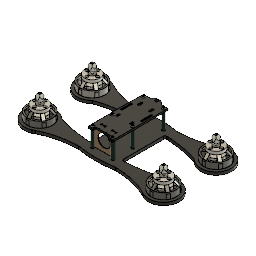
Carbon Fibre Drone Exam v2 (Autodesk Fusion 360 design; units mm, degrees)
Autodesk Fusion 360 part; units mm, degrees
note: some values were not read from the file. Chosen so that the rebuilt part matches the saved one: which bodies a step acts on; which face or edge a step refers to. Set by a fixed rule: which sketch regions a step uses.
(part 1 of 2)
sketch "Sketch1" plane through (0, 0, 0) normal (0, 1, 0) x (1, 0, 0) in component "Component"
  line L0 (50, -100) -> (-50, 100) construction
  line L1 (-50, -100) -> (50, 100) construction
  line L2 (199.7933, 69.8317) -> (-200.2067, 99.8317) construction
  line L3 (-200.2067, 69.8317) -> (199.7933, 99.8317) construction
  line L4 (-150, 0) -> (150, 0) construction
  line L5 (-200.2067, -99.8317) -> (-200.2067, -84.8317) construction
  line L6 (0, 150) -> (0, -200) construction
  spline S0 degree 5 poles (-164.8811, -49.4467) (-163.5288, -50.018) (-160.7538, -51.1452) (-156.3792, -52.7897) (-150.1158, -54.8884) (-141.5256, -57.3456) (-132.1253, -59.6259) (-121.8831, -61.7224) (-110.8317, -63.6422) (-99.042, -65.4008) (-86.5906, -67.0149) (-76.1522, -68.202) (-68.0735, -69.0377) (-62.5785, -69.571) (-59.8037, -69.8317) knots 0 0 0 0 0 0 0.1 0.2 0.3 0.4 0.5 0.6 0.7 0.8 0.9 1 1 1 1 1 1
  spline S1 degree 5 poles (-179.5589, -130.3693) (-177.6465, -129.2803) (-173.7784, -127.1456) (-167.8467, -124.0728) (-159.6742, -120.2387) (-148.9906, -115.9128) (-137.8023, -112.0905) (-126.0755, -108.8054) (-113.8059, -106.0617) (-101.0284, -103.8246) (-87.7873, -102.05) (-76.857, -100.967) (-68.4818, -100.3317) (-62.8209, -99.9855) (-59.9711, -99.8317) knots 0 0 0 0 0 0 0.1 0.2 0.3 0.4 0.5 0.6 0.7 0.8 0.9 1 1 1 1 1 1
  spline S2 degree 5 poles (-179.5589, 130.3693) (-177.6465, 129.2803) (-173.7784, 127.1456) (-167.8467, 124.0728) (-159.6742, 120.2387) (-148.9906, 115.9128) (-137.8023, 112.0905) (-126.0755, 108.8054) (-113.8059, 106.0617) (-101.0284, 103.8246) (-87.7873, 102.05) (-76.857, 100.967) (-68.4818, 100.3317) (-62.8209, 99.9855) (-59.9711, 99.8317) knots 0 0 0 0 0 0 0.1 0.2 0.3 0.4 0.5 0.6 0.7 0.8 0.9 1 1 1 1 1 1
  line L7 (-190.3068, -136.4894) -> (-168.8109, -124.2492)
  line L8 (-73.9023, -100.583) -> (-46.0398, -99.0805)
  line L9 (-190.3068, 136.4894) -> (-168.8109, 124.2492)
  line L10 (-73.9023, 100.583) -> (-46.0398, 99.0805)
  spline S3 degree 5 poles (-164.8811, 49.4467) (-163.5288, 50.018) (-160.7538, 51.1452) (-156.3792, 52.7897) (-150.1158, 54.8884) (-141.5256, 57.3456) (-132.1253, 59.6259) (-121.8831, 61.7224) (-110.8317, 63.6422) (-99.042, 65.4008) (-86.5906, 67.0149) (-76.1522, 68.202) (-68.0735, 69.0377) (-62.5785, 69.571) (-59.8037, 69.8317) knots 0 0 0 0 0 0 0.1 0.2 0.3 0.4 0.5 0.6 0.7 0.8 0.9 1 1 1 1 1 1
  line L11 (-173.4718, -45.817) -> (-156.2903, -53.0763)
  line L12 (-72.3823, -68.6499) -> (-47.2251, -71.0135)
  line L13 (-173.4718, 45.817) -> (-156.2903, 53.0763)
  line L14 (-72.3823, 68.6499) -> (-47.2251, 71.0135)
  spline S4 degree 5 poles (164.8811, 49.4467) (163.5288, 50.018) (160.7538, 51.1452) (156.3792, 52.7897) (150.1158, 54.8884) (141.5256, 57.3456) (132.1253, 59.6259) (121.8831, 61.7224) (110.8317, 63.6422) (99.042, 65.4008) (86.5906, 67.0149) (76.1522, 68.202) (68.0735, 69.0377) (62.5785, 69.571) (59.8037, 69.8317) knots 0 0 0 0 0 0 0.1 0.2 0.3 0.4 0.5 0.6 0.7 0.8 0.9 1 1 1 1 1 1
  line L15 (173.4718, 45.817) -> (156.2903, 53.0763)
  line L16 (72.3823, 68.6499) -> (47.2251, 71.0135)
  spline S5 degree 5 poles (179.5589, -130.3693) (177.6465, -129.2803) (173.7784, -127.1456) (167.8467, -124.0728) (159.6742, -120.2387) (148.9906, -115.9128) (137.8023, -112.0905) (126.0755, -108.8054) (113.8059, -106.0617) (101.0284, -103.8246) (87.7873, -102.05) (76.857, -100.967) (68.4818, -100.3317) (62.8209, -99.9855) (59.9711, -99.8317) knots 0 0 0 0 0 0 0.1 0.2 0.3 0.4 0.5 0.6 0.7 0.8 0.9 1 1 1 1 1 1
  line L17 (190.3068, -136.4894) -> (168.8109, -124.2492)
  line L18 (73.9023, -100.583) -> (46.0398, -99.0805)
  spline S6 degree 5 poles (164.8811, -49.4467) (163.5288, -50.018) (160.7538, -51.1452) (156.3792, -52.7897) (150.1158, -54.8884) (141.5256, -57.3456) (132.1253, -59.6259) (121.8831, -61.7224) (110.8317, -63.6422) (99.042, -65.4008) (86.5906, -67.0149) (76.1522, -68.202) (68.0735, -69.0377) (62.5785, -69.571) (59.8037, -69.8317) knots 0 0 0 0 0 0 0.1 0.2 0.3 0.4 0.5 0.6 0.7 0.8 0.9 1 1 1 1 1 1
  line L19 (173.4718, -45.817) -> (156.2903, -53.0763)
  line L20 (72.3823, -68.6499) -> (47.2251, -71.0135)
  spline S7 degree 5 poles (179.5589, 130.3693) (177.6465, 129.2803) (173.7784, 127.1456) (167.8467, 124.0728) (159.6742, 120.2387) (148.9906, 115.9128) (137.8023, 112.0905) (126.0755, 108.8054) (113.8059, 106.0617) (101.0284, 103.8246) (87.7873, 102.05) (76.857, 100.967) (68.4818, 100.3317) (62.8209, 99.9855) (59.9711, 99.8317) knots 0 0 0 0 0 0 0.1 0.2 0.3 0.4 0.5 0.6 0.7 0.8 0.9 1 1 1 1 1 1
  line L21 (190.3068, 136.4894) -> (168.8109, 124.2492)
  line L22 (73.9023, 100.583) -> (46.0398, 99.0805)
  spline S8 degree 5 poles (-59.9711, 99.8317) (-57.5722, 100.2237) (-52.7745, 100.9735) (-45.578, 101.9954) (-35.9826, 103.1493) (-23.9884, 104.2199) (-11.9942, 104.8857) (0, 105.1137) (11.9942, 104.8857) (23.9884, 104.2199) (35.9826, 103.1493) (45.578, 101.9954) (52.7745, 100.9735) (57.5722, 100.2237) (59.9711, 99.8317) knots 0 0 0 0 0 0 0.1 0.2 0.3 0.4 0.5 0.6 0.7 0.8 0.9 1 1 1 1 1 1
  spline S9 degree 5 poles (-59.9711, -99.8317) (-57.5722, -100.2237) (-52.7745, -100.9735) (-45.578, -101.9954) (-35.9826, -103.1493) (-23.9884, -104.2199) (-11.9942, -104.8857) (0, -105.1137) (11.9942, -104.8857) (23.9884, -104.2199) (35.9826, -103.1493) (45.578, -101.9954) (52.7745, -100.9735) (57.5722, -100.2237) (59.9711, -99.8317) knots 0 0 0 0 0 0 0.1 0.2 0.3 0.4 0.5 0.6 0.7 0.8 0.9 1 1 1 1 1 1
  line L23 (-72.1535, 97.8409) -> (-47.7886, 101.8226)
  line L24 (47.7882, 101.8225) -> (72.1539, 97.841)
  line L25 (-72.1535, -97.8409) -> (-47.7886, -101.8226)
  line L26 (47.7882, -101.8225) -> (72.1539, -97.841)
  line L27 (50, -99.8317) -> (50, -100)
  line L28 (-50, -100) -> (-50, -99.8317)
  line L29 (-50, -99.8317) -> (-49.9159, -99.8317)
  line L30 (49.9159, -99.8317) -> (50, -99.8317)
  arc A0 (-164.8811, -49.4467) -> (-173.0625, -126.8222) centre (-200.2067, -84.8317) ccw
  arc A1 (173.0625, -126.8222) -> (164.8811, -49.4467) centre (200.2067, -84.8317) ccw
  line L31 (59.8037, -69.8317) -> (55, -69.8317)
  line L32 (-55, -69.8317) -> (-59.8037, -69.8317)
  arc A2 (-173.0625, 126.8222) -> (-164.8811, 49.4467) centre (-200.2067, 84.8317) ccw
  line L33 (-50, 99.8317) -> (-49.9159, 99.8317)
  line L34 (-55, 69.8317) -> (-59.8037, 69.8317)
  line L35 (49.9159, 99.8317) -> (50, 99.8317)
  line L36 (50, 100) -> (50, 99.8317)
  line L37 (50, 64.8317) -> (50, -64.8317)
  line L38 (59.8037, 69.8317) -> (55, 69.8317)
  arc A3 (164.8811, 49.4467) -> (173.0625, 126.8221) centre (200.2067, 84.8317) ccw
  line L39 (-50, -64.8317) -> (-50, 64.8317)
  line L40 (-50, 99.8317) -> (-50, 100)
  arc A4 (-50, 64.8317) -> (-55, 69.8317) centre (-55, 64.8317) ccw
  arc A5 (-55, -69.8317) -> (-50, -64.8317) centre (-55, -64.8317) ccw
  arc A6 (50, -64.8317) -> (55, -69.8317) centre (55, -64.8317) ccw
  arc A7 (55, 69.8317) -> (50, 64.8317) centre (55, 64.8317) ccw
  point P0 (-0.2067, 84.8317)
  point P1 (-130, -60)
  point P2 (-130, -110)
  point P3 (-130, 110)
  point P4 (-130, 60)
  point P5 (130, -60)
  point P6 (130, 60)
  point P7 (130, -110)
  point P8 (130, 110)
  point P9 (0, 105)
  point P10 (0, -105)
  dimension "d1" = 100
  dimension "d2" = 200
  dimension "d3" = 400
  dimension "d4" = 30
  dimension "d5" = 15
  dimension "d6" = 100
  dimension "d7" = 5
  dimension "d8" = 5
  dimension "d9" = 5
  dimension "d10" = 5
  constraint parallel L28 L36
  constraint coincident L0 origin
  constraint coincident L1 origin
  constraint coincident L2 P0
  constraint coincident L3 P0
  constraint perpendicular L4 L36
  constraint symmetric L2.end L4 L5.start
  constraint coincident L5.end A0.centre
  constraint symmetric L4 A0 A2
  constraint symmetric L6 A0 A1
  constraint symmetric L6 A2 A3
  constraint coincident S1.start A0
  constraint midpoint S1.start L7
  constraint midpoint S1.end L8
  constraint midpoint S0.start L11
  constraint midpoint S0.end L12
  constraint symmetric L4 S0.start S3.start
  constraint symmetric L4 P1 P4
  constraint symmetric L4 S0.end S3.end
  constraint symmetric L4 S1.start S2.start
  constraint symmetric L4 P2 P3
  constraint symmetric L4 S1.end S2.end
  constraint symmetric L4 L7.start L9.start
  constraint symmetric L4 L7.end L9.end
  constraint symmetric L4 L8.start L10.start
  constraint symmetric L4 L8.end L10.end
  constraint symmetric L4 L11.start L13.start
  constraint symmetric L4 L11.end L13.end
  constraint symmetric L4 L12.start L14.start
  constraint symmetric L4 L12.end L14.end
  constraint symmetric L6 S0.start S6.start
  constraint symmetric L6 P1 P5
  constraint symmetric L6 S0.end S6.end
  constraint symmetric L6 S1.start S5.start
  constraint symmetric L6 P2 P7
  constraint symmetric L6 S1.end S5.end
  constraint symmetric L6 S2.start S7.start
  constraint symmetric L6 P3 P8
  constraint symmetric L6 S2.end S7.end
  constraint symmetric L6 L7.start L17.start
  constraint symmetric L6 L7.end L17.end
  constraint symmetric L6 L8.start L18.start
  constraint symmetric L6 L8.end L18.end
  constraint symmetric L6 L9.start L21.start
  constraint symmetric L6 L9.end L21.end
  constraint symmetric L6 L10.start L22.start
  constraint symmetric L6 L10.end L22.end
  constraint symmetric L6 S3.start S4.start
  constraint symmetric L6 P4 P6
  constraint symmetric L6 S3.end S4.end
  constraint symmetric L6 L11.start L19.start
  constraint symmetric L6 L11.end L19.end
  constraint symmetric L6 L12.start L20.start
  constraint symmetric L6 L12.end L20.end
  constraint symmetric L6 L13.start L15.start
  constraint symmetric L6 L13.end L15.end
  constraint symmetric L6 L14.start L16.start
  constraint symmetric L6 L14.end L16.end
  constraint coincident L6 P9
  constraint midpoint S2.end L23
  constraint midpoint S7.end L24
  constraint symmetric L4 S2.end S1.end
  constraint symmetric L4 S7.end S5.end
  constraint symmetric L4 P9 P10
  constraint symmetric L4 L23.start L25.start
  constraint symmetric L4 L23.end L25.end
  constraint symmetric L4 L24.start L26.start
  constraint symmetric L4 L24.end L26.end
  constraint coincident L27.start L36
  constraint collinear L27 L36
  constraint collinear L28 L39
  constraint coincident L0 L30.start
  constraint collinear L29 L30
  constraint coincident L1 L29.end
  constraint coincident S1 A0.end
  constraint coincident S5 A1.start
  constraint collinear L31 L32
  constraint coincident L1 L35.start
  constraint collinear L33 L35
  constraint coincident S2 A2.start
  constraint coincident L0 L33.end
  constraint coincident L33.start L39
  constraint collinear L36 L37
  constraint coincident S7 A3.end
  constraint collinear L39 L40
  constraint tangent L34 A4
  constraint tangent L39 A4
  constraint tangent L32 A5
  constraint tangent L39 A5
  constraint tangent L37 A6
  constraint tangent L31 A6
  constraint tangent L37 A7
  constraint tangent L38 A7
  measures "d1" distance of L0.end L1.end
  measures "d2" distance of L1.start L0.end
  measures "d3" distance of L2.end L3.end
  measures "d4" distance of L3.start L2.end
  measures "d5" distance of L5.start L5.end
  measures "d6" diameter of A0
  measures "d7" radius of A4
  measures "d8" radius of A5
  measures "d9" radius of A6
  measures "d10" radius of A7
extrude "Extrude1" add sketch "Sketch1" along normal blind 10 contours S0 S1 S2 S3 S4 S5 S6 S7 S8 S9 A0 A1 L31 L32 A2 L34 L37 L38 A3 L39 A4 A5 A6 A7 makes body 1 in component "Component"
sketch "Sketch1 (2)" plane through (0, 10, 0) normal (0, 1, 0) x (-1, 0, 0) in component "Component'"
  arc A0 (-164.8811, -49.4467) -> (-179.5589, -130.3693) centre (-200.2067, -84.8317) ccw
  spline S0 degree 5 poles (-179.5589, -130.3693) (-178.279, -129.6405) (-176.9894, -128.9214) (-175.6902, -128.2119) (-174.3812, -127.5121) (-173.0625, -126.8221) knots 0 0 0 0 0 0 0.066925 0.066925 0.066925 0.066925 0.066925 0.066925
  spline S1 degree 5 poles (-173.0625, -126.8221) (-172.4108, -126.4811) (-169.779, -125.1187) (-165.1015, -122.8003) (-158.2442, -119.6597) (-148.9906, -115.9128) (-137.8023, -112.0905) (-126.0755, -108.8054) (-113.8059, -106.0617) (-101.0284, -103.8246) (-87.7873, -102.05) (-76.857, -100.967) (-68.4818, -100.3317) (-62.8209, -99.9855) (-59.9711, -99.8317) knots 0.066925 0.066925 0.066925 0.066925 0.066925 0.066925 0.1 0.2 0.3 0.4 0.5 0.6 0.7 0.8 0.9 1 1 1 1 1 1
  spline S2 degree 5 poles (-59.9711, -99.8317) (-57.5722, -100.2237) (-52.7745, -100.9735) (-45.578, -101.9954) (-35.9826, -103.1493) (-23.9884, -104.2199) (-11.9942, -104.8857) (0, -105.1137) (11.9942, -104.8857) (23.9884, -104.2199) (35.9826, -103.1493) (45.578, -101.9954) (52.7745, -100.9735) (57.5722, -100.2237) (59.9711, -99.8317) knots -1 -1 -1 -1 -1 -1 -0.9 -0.8 -0.7 -0.6 -0.5 -0.4 -0.3 -0.2 -0.1 0 0 0 0 0 0
  spline S3 degree 5 poles (59.9711, -99.8317) (62.8209, -99.9855) (68.4818, -100.3317) (76.857, -100.967) (87.7873, -102.05) (101.0284, -103.8246) (113.8059, -106.0617) (126.0755, -108.8054) (137.8023, -112.0905) (148.9906, -115.9128) (158.2442, -119.6597) (165.1015, -122.8003) (169.779, -125.1187) (172.4108, -126.4811) (173.0625, -126.8222) knots -1 -1 -1 -1 -1 -1 -0.9 -0.8 -0.7 -0.6 -0.5 -0.4 -0.3 -0.2 -0.1 -0.066925 -0.066925 -0.066925 -0.066925 -0.066925 -0.066925
  spline S4 degree 5 poles (173.0625, -126.8222) (174.3813, -127.5122) (175.6902, -128.2119) (176.9894, -128.9214) (178.279, -129.6405) (179.5589, -130.3693) knots -0.066925 -0.066925 -0.066925 -0.066925 -0.066925 -0.066925 0 0 0 0 0 0
  arc A1 (179.5589, -130.3693) -> (164.8811, -49.4467) centre (200.2067, -84.8317) ccw
  spline S5 degree 5 poles (164.8811, -49.4467) (163.5288, -50.018) (160.7538, -51.1452) (156.3792, -52.7897) (150.1158, -54.8884) (141.5256, -57.3456) (132.1253, -59.6259) (121.8831, -61.7224) (110.8317, -63.6422) (99.042, -65.4008) (86.5906, -67.0149) (76.1522, -68.202) (68.0735, -69.0377) (62.5785, -69.571) (59.8037, -69.8317) knots 0 0 0 0 0 0 0.1 0.2 0.3 0.4 0.5 0.6 0.7 0.8 0.9 1 1 1 1 1 1
  line L0 (59.8037, -69.8317) -> (55, -69.8317)
  arc A2 (50, -64.8317) -> (55, -69.8317) centre (55, -64.8317) ccw
  line L1 (50, -64.8317) -> (50, 64.8317)
  arc A3 (55, 69.8317) -> (50, 64.8317) centre (55, 64.8317) ccw
  line L2 (55, 69.8317) -> (59.8037, 69.8317)
  spline S6 degree 5 poles (59.8037, 69.8317) (62.5785, 69.571) (68.0735, 69.0377) (76.1522, 68.202) (86.5906, 67.0149) (99.042, 65.4008) (110.8317, 63.6422) (121.8831, 61.7224) (132.1253, 59.6259) (141.5256, 57.3456) (150.1158, 54.8884) (156.3792, 52.7897) (160.7538, 51.1452) (163.5288, 50.018) (164.8811, 49.4467) knots -1 -1 -1 -1 -1 -1 -0.9 -0.8 -0.7 -0.6 -0.5 -0.4 -0.3 -0.2 -0.1 0 0 0 0 0 0
  arc A4 (164.8811, 49.4467) -> (179.5589, 130.3693) centre (200.2067, 84.8317) ccw
  spline S7 degree 5 poles (179.5589, 130.3693) (178.279, 129.6405) (176.9894, 128.9214) (175.6902, 128.2119) (174.3813, 127.5122) (173.0625, 126.8222) knots 0 0 0 0 0 0 0.066925 0.066925 0.066925 0.066925 0.066925 0.066925
  spline S8 degree 5 poles (173.0625, 126.8222) (172.4108, 126.4811) (169.779, 125.1187) (165.1015, 122.8003) (158.2442, 119.6597) (148.9906, 115.9128) (137.8023, 112.0905) (126.0755, 108.8054) (113.8059, 106.0617) (101.0284, 103.8246) (87.7873, 102.05) (76.857, 100.967) (68.4818, 100.3317) (62.8209, 99.9855) (59.9711, 99.8317) knots 0.066925 0.066925 0.066925 0.066925 0.066925 0.066925 0.1 0.2 0.3 0.4 0.5 0.6 0.7 0.8 0.9 1 1 1 1 1 1
  spline S9 degree 5 poles (59.9711, 99.8317) (57.5722, 100.2237) (52.7745, 100.9735) (45.578, 101.9954) (35.9826, 103.1493) (23.9884, 104.2199) (11.9942, 104.8857) (0, 105.1137) (-11.9942, 104.8857) (-23.9884, 104.2199) (-35.9826, 103.1493) (-45.578, 101.9954) (-52.7745, 100.9735) (-57.5722, 100.2237) (-59.9711, 99.8317) knots 0 0 0 0 0 0 0.1 0.2 0.3 0.4 0.5 0.6 0.7 0.8 0.9 1 1 1 1 1 1
  spline S10 degree 5 poles (-59.9711, 99.8317) (-62.8209, 99.9855) (-68.4818, 100.3317) (-76.857, 100.967) (-87.7873, 102.05) (-101.0284, 103.8246) (-113.8059, 106.0617) (-126.0755, 108.8054) (-137.8023, 112.0905) (-148.9906, 115.9128) (-158.2442, 119.6597) (-165.1015, 122.8003) (-169.779, 125.1187) (-172.4108, 126.4811) (-173.0625, 126.8222) knots -1 -1 -1 -1 -1 -1 -0.9 -0.8 -0.7 -0.6 -0.5 -0.4 -0.3 -0.2 -0.1 -0.066925 -0.066925 -0.066925 -0.066925 -0.066925 -0.066925
  spline S11 degree 5 poles (-173.0625, 126.8222) (-174.3813, 127.5122) (-175.6902, 128.2119) (-176.9894, 128.9214) (-178.279, 129.6405) (-179.5589, 130.3693) knots -0.066925 -0.066925 -0.066925 -0.066925 -0.066925 -0.066925 0 0 0 0 0 0
  arc A5 (-179.5589, 130.3693) -> (-164.8811, 49.4467) centre (-200.2067, 84.8317) ccw
  spline S12 degree 5 poles (-164.8811, 49.4467) (-163.5288, 50.018) (-160.7538, 51.1452) (-156.3792, 52.7897) (-150.1158, 54.8884) (-141.5256, 57.3456) (-132.1253, 59.6259) (-121.8831, 61.7224) (-110.8317, 63.6422) (-99.042, 65.4008) (-86.5906, 67.0149) (-76.1522, 68.202) (-68.0735, 69.0377) (-62.5785, 69.571) (-59.8037, 69.8317) knots 0 0 0 0 0 0 0.1 0.2 0.3 0.4 0.5 0.6 0.7 0.8 0.9 1 1 1 1 1 1
  line L3 (-59.8037, 69.8317) -> (-55, 69.8317)
  arc A6 (-50, 64.8317) -> (-55, 69.8317) centre (-55, 64.8317) ccw
  line L4 (-50, 64.8317) -> (-50, -64.8317)
  arc A7 (-55, -69.8317) -> (-50, -64.8317) centre (-55, -64.8317) ccw
  line L5 (-55, -69.8317) -> (-59.8037, -69.8317)
  spline S13 degree 5 poles (-59.8037, -69.8317) (-62.5785, -69.571) (-68.0735, -69.0377) (-76.1522, -68.202) (-86.5906, -67.0149) (-99.042, -65.4008) (-110.8317, -63.6422) (-121.8831, -61.7224) (-132.1253, -59.6259) (-141.5256, -57.3456) (-150.1158, -54.8884) (-156.3792, -52.7897) (-160.7538, -51.1452) (-163.5288, -50.018) (-164.8811, -49.4467) knots -1 -1 -1 -1 -1 -1 -0.9 -0.8 -0.7 -0.6 -0.5 -0.4 -0.3 -0.2 -0.1 0 0 0 0 0 0
  line L6 (40, 88) -> (40, -90)
  line L7 (-40, -90) -> (-40, 88)
  line L8 (-40, 90) -> (40, -90) construction
  line L9 (40, 90) -> (-40, -90) construction
  line L10 (23, 79.4003) -> (-23, 79.4003)
  line L11 (-25, 81.4003) -> (-25, 88)
  line L12 (25, 88) -> (25, 81.4003)
  circle A8 centre (33, 82) radius 5
  line L13 (-38, 90) -> (-27, 90)
  line L14 (27, 90) -> (38, 90)
  arc A9 (23, 79.4003) -> (25, 81.4003) centre (23, 81.4003) ccw
  arc A10 (27, 90) -> (25, 88) centre (27, 88) ccw
  arc A11 (40, 88) -> (38, 90) centre (38, 88) ccw
  arc A12 (-25, 81.4003) -> (-23, 79.4003) centre (-23, 81.4003) ccw
  arc A13 (-25, 88) -> (-27, 90) centre (-27, 88) ccw
  arc A14 (-38, 90) -> (-40, 88) centre (-38, 88) ccw
  line L15 (0, 0) -> (0, 150)
  line L16 (0, 150) -> (0, 0)
  line L17 (0, 0) -> (0, -150)
  circle A15 centre (-33, 82) radius 5
  line L18 (150, 0) -> (-150, 0)
  line L19 (150, 50) -> (-150, 50)
  circle A16 centre (33, 18) radius 5
  circle A17 centre (-33, 18) radius 5
  circle A18 centre (33, -82) radius 5
  circle A19 centre (-33, -82) radius 5
  line L20 (11.2, 59) -> (10.8383, 59)
  line L21 (10.0383, 59.8) -> (10.0383, 64.2284)
  line L22 (10.8383, 65.0284) -> (11.2, 65.0284)
  line L23 (24, 59.2) -> (24.0338, 59.2)
  line L24 (24.0338, 65.0284) -> (24, 65.0284)
  line L25 (24.8, 64.2284) -> (24.8, 60)
  line L26 (23.2338, 61.1579) -> (12, 61.1579)
  line L27 (12, 63.1245) -> (23.2338, 63.1245)
  line L28 (23.2338, 60) -> (23.2338, 61.1579)
  line L29 (23.2338, 63.1245) -> (23.2338, 64.2284)
  line L30 (12, 64.2284) -> (12, 63.1245)
  line L31 (12, 61.1579) -> (12, 59.8)
  arc A20 (23.2338, 60) -> (24.0338, 59.2) centre (24.0338, 60) ccw
  arc A21 (24, 59.2) -> (24.8, 60) centre (24, 60) ccw
  arc A22 (24.8, 64.2284) -> (24, 65.0284) centre (24, 64.2284) ccw
  arc A23 (24.0338, 65.0284) -> (23.2338, 64.2284) centre (24.0338, 64.2284) ccw
  arc A24 (11.2, 59) -> (12, 59.8) centre (11.2, 59.8) ccw
  arc A25 (10.0383, 59.8) -> (10.8383, 59) centre (10.8383, 59.8) ccw
  arc A26 (12, 64.2284) -> (11.2, 65.0284) centre (11.2, 64.2284) ccw
  arc A27 (10.8383, 65.0284) -> (10.0383, 64.2284) centre (10.8383, 64.2284) ccw
  line L32 (18.3125, -64.8317) -> (18, -64.8317)
  line L33 (15, -61.8317) -> (15, -53)
  line L34 (18, -50) -> (18.3125, -50)
  line L35 (21.3125, -53) -> (21.3125, -61.8317)
  line L36 (35, -45) -> (30, -45)
  line L37 (30, -45) -> (30, -10)
  line L38 (30, -10) -> (35, -10)
  line L39 (35, -10) -> (35, -45)
  arc A28 (15, -61.8317) -> (18, -64.8317) centre (18, -61.8317) ccw
  arc A29 (18.3125, -64.8317) -> (21.3125, -61.8317) centre (18.3125, -61.8317) ccw
  arc A30 (21.3125, -53) -> (18.3125, -50) centre (18.3125, -53) ccw
  arc A31 (18, -50) -> (15, -53) centre (18, -53) ccw
  line L40 (-30, -45) -> (-30, -10)
  line L41 (-35, -10) -> (-35, -45)
  line L42 (-35, -45) -> (-30, -45)
  line L43 (-30, -10) -> (-35, -10)
  line L44 (-15, -61.8317) -> (-15, -53)
  arc A32 (-15, -53) -> (-18, -50) centre (-18, -53) ccw
  arc A33 (-18.3125, -50) -> (-21.3125, -53) centre (-18.3125, -53) ccw
  line L45 (-21.3125, -53) -> (-21.3125, -61.8317)
  arc A34 (-21.3125, -61.8317) -> (-18.3125, -64.8317) centre (-18.3125, -61.8317) ccw
  arc A35 (-18, -64.8317) -> (-15, -61.8317) centre (-18, -61.8317) ccw
  line L46 (-18.3125, -64.8317) -> (-18, -64.8317)
  line L47 (-18, -50) -> (-18.3125, -50)
  line L48 (-12, 63.1245) -> (-23.2338, 63.1245)
  line L49 (-23.2338, 61.1579) -> (-12, 61.1579)
  line L50 (-24.8, 64.2284) -> (-24.8, 60)
  arc A36 (-23.2338, 64.2284) -> (-24.0338, 65.0284) centre (-24.0338, 64.2284) ccw
  arc A37 (-24, 65.0284) -> (-24.8, 64.2284) centre (-24, 64.2284) ccw
  line L51 (-23.2338, 63.1245) -> (-23.2338, 64.2284)
  line L52 (-23.2338, 60) -> (-23.2338, 61.1579)
  arc A38 (-24.8, 60) -> (-24, 59.2) centre (-24, 60) ccw
  arc A39 (-24.0338, 59.2) -> (-23.2338, 60) centre (-24.0338, 60) ccw
  line L53 (-10.0383, 59.8) -> (-10.0383, 64.2284)
  line L54 (-12, 64.2284) -> (-12, 63.1245)
  arc A40 (-11.2, 65.0284) -> (-12, 64.2284) centre (-11.2, 64.2284) ccw
  line L55 (-12, 61.1579) -> (-12, 59.8)
  arc A41 (-12, 59.8) -> (-11.2, 59) centre (-11.2, 59.8) ccw
  line L56 (-11.2, 59) -> (-10.8383, 59)
  arc A42 (-10.8383, 59) -> (-10.0383, 59.8) centre (-10.8383, 59.8) ccw
  arc A43 (-10.0383, 64.2284) -> (-10.8383, 65.0284) centre (-10.8383, 64.2284) ccw
  line L57 (-10.8383, 65.0284) -> (-11.2, 65.0284)
  line L58 (25, 5) -> (20, 5)
  line L59 (20, 5) -> (20, 15)
  line L60 (20, 15) -> (25, 15)
  line L61 (25, 15) -> (25, 5)
  line L62 (-20, 5) -> (-20, 15)
  line L63 (-25, 5) -> (-20, 5)
  line L64 (-25, 15) -> (-25, 5)
  line L65 (-20, 15) -> (-25, 15)
  arc A44 (-16.3, -92.0308) -> (16.3, -92.0308) centre (0, -80) ccw
  line L66 (40, -90) -> (20.3229, -90)
  line L67 (-20.3229, -90) -> (-40, -90)
  arc A45 (20.3229, -90) -> (16.3, -92.0308) centre (20.3229, -95) ccw
  arc A46 (-16.3, -92.0308) -> (-20.3229, -90) centre (-20.3229, -95) ccw
  circle A47 centre (0, -93.2666) radius 5
  point P0 (-33, -82)
  dimension "d13" = 10
  dimension "d14" = 2
  dimension "d15" = 2
  dimension "d16" = 2
  dimension "d17" = 2
  dimension "d18" = 2
  dimension "d19" = 2
  dimension "d20" = 10
  dimension "d21" = 0.8
  dimension "d22" = 0.8
  dimension "d23" = 0.8
  dimension "d24" = 0.8
  dimension "d25" = 0.8
  dimension "d26" = 0.8
  dimension "d27" = 0.8
  dimension "d28" = 0.8
  dimension "d29" = 3
  dimension "d30" = 3
  dimension "d31" = 3
  dimension "d32" = 3
  dimension "d33" = 5
  dimension "d34" = 5
  dimension "d37" = 10
  constraint horizontal L13
  constraint perpendicular L6 L13
  constraint parallel L13 L66
  constraint parallel L6 L7
  constraint coincident L8 L15.start
  constraint coincident L9 L15.start
  constraint coincident L15.start L16.end
  constraint horizontal L10
  constraint vertical L11
  constraint vertical L12
  constraint collinear L13 L14
  constraint tangent L12 A9
  constraint tangent L10 A9
  constraint tangent L12 A10
  constraint tangent L14 A10
  constraint coincident L9.start L6
  constraint coincident L9.start L14
  constraint tangent L6 A11
  constraint tangent L14 A11
  constraint tangent L10 A12
  constraint tangent L11 A12
  constraint tangent L11 A13
  constraint tangent L13 A13
  constraint coincident L8.start L13
  constraint coincident L8.start L7
  constraint tangent L13 A14
  constraint tangent L7 A14
  constraint perpendicular L10 L15
  constraint parallel L15 L16
  constraint perpendicular L17 L66
  constraint symmetric A8 L16 A15
  constraint perpendicular L4 L18
  constraint perpendicular L4 L19
  constraint symmetric A8 L19 A16
  constraint symmetric A15 L19 A17
  constraint symmetric A8 L18 A18
  constraint symmetric A15.centre L18 P0
  constraint coincident P0 A19.centre
  constraint coincident L17 A44.centre
  constraint horizontal L27
  constraint horizontal L20
  constraint vertical L21
  constraint horizontal L22
  constraint vertical L30
  constraint horizontal L23
  constraint vertical L28
  constraint horizontal L24
  constraint vertical L25
  constraint coincident L27.end L28
  constraint collinear L28 L29
  constraint collinear L30 L31
  constraint tangent L28 A20
  constraint tangent L23 A20
  constraint tangent L23 A21
  constraint tangent L25 A21
  constraint tangent L25 A22
  constraint tangent L24 A22
  constraint tangent L29 A23
  constraint tangent L24 A23
  constraint tangent L31 A24
  constraint tangent L20 A24
  constraint tangent L21 A25
  constraint tangent L20 A25
  constraint tangent L30 A26
  constraint tangent L22 A26
  constraint tangent L22 A27
  constraint tangent L21 A27
  constraint horizontal L32
  constraint vertical L33
  constraint horizontal L34
  constraint vertical L35
  constraint horizontal L36
  constraint vertical L37
  constraint horizontal L38
  constraint vertical L39
  constraint tangent L32 A28
  constraint tangent L33 A28
  constraint tangent L32 A29
  constraint tangent L35 A29
  constraint tangent L35 A30
  constraint tangent L34 A30
  constraint tangent L33 A31
  constraint tangent L34 A31
  constraint symmetric L15 L26.start L49.start
  constraint symmetric L15 L27.end L48.end
  constraint symmetric L15 L27.start L48.start
  constraint symmetric L15 L26.end L49.end
  constraint symmetric L15 L28.start L52.start
  constraint symmetric L15 L23.end A39.start
  constraint symmetric L15 A20 A39
  constraint symmetric L15 L23.start A38.end
  constraint symmetric L15 L25.end L50.end
  constraint symmetric L15 A21 A38
  constraint symmetric L15 L25.start L50.start
  constraint symmetric L15 L24.end A37.start
  constraint symmetric L15 A22 A37
  constraint symmetric L15 L29.end A36.start
  constraint symmetric L15 L24.start A36.end
  constraint symmetric L15 A23 A36
  constraint symmetric L15 L31.end L55.end
  constraint symmetric L15 L20.start A41.end
  constraint symmetric L15 A24 A41
  constraint symmetric L15 L21.start L53.start
  constraint symmetric L15 L20.end L56.end
  constraint symmetric L15 A25 A42
  constraint symmetric L15 L30.start L54.start
  constraint symmetric L15 L22.end A40.start
  constraint symmetric L15 A26 A40
  constraint symmetric L15 L22.start A43.end
  constraint symmetric L15 L21.end L53.end
  constraint symmetric L15 A27 A43
  constraint symmetric L15 L36.start L41.end
  constraint symmetric L15 L36.end L40.start
  constraint symmetric L15 L37.end L40.end
  constraint symmetric L15 L38.end L41.start
  constraint symmetric L15 L32.end A35.start
  constraint symmetric L15 L33.start L44.start
  constraint symmetric L15 A28 A35
  constraint symmetric L15 L32.start A34.end
  constraint symmetric L15 L35.end L45.end
  constraint symmetric L15 A29 A34
  constraint symmetric L15 L35.start A33.end
  constraint symmetric L15 L34.end A33.start
  constraint symmetric L15 A30 A33
  constraint symmetric L15 L33.end L44.end
  constraint symmetric L15 L34.start A32.end
  constraint symmetric L15 A31 A32
  constraint horizontal L58
  constraint vertical L59
  constraint horizontal L60
  constraint vertical L61
  constraint symmetric L15 L58.start L63.start
  constraint symmetric L15 L58.end L62.start
  constraint symmetric L15 L59.end L62.end
  constraint symmetric L15 L60.end L64.start
  constraint collinear L66 L67
  constraint tangent L66 A45
  constraint tangent A44 A45
  constraint tangent A44 A46
  constraint tangent L67 A46
  constraint coincident L17 A47.centre
  measures "d13" diameter of A8
  measures "d14" radius of A9
  measures "d15" radius of A10
  measures "d16" radius of A11
  measures "d17" radius of A12
  measures "d18" radius of A13
  measures "d19" radius of A14
  measures "d20" diameter of A19
  measures "d21" radius of A20
  measures "d22" radius of A21
  measures "d23" radius of A22
  measures "d24" radius of A23
  measures "d25" radius of A24
  measures "d26" radius of A25
  measures "d27" radius of A26
  measures "d28" radius of A27
  measures "d29" radius of A28
  measures "d30" radius of A29
  measures "d31" radius of A30
  measures "d32" radius of A31
  measures "d33" radius of A45
  measures "d34" radius of A46
  measures "d37" diameter of A47
extrude "Extrude2" add sketch "Sketch1 (2)" along normal blind 58 separate body contours L20 L21 L22 L23 L24 L25 L26 L27 L28 L29 L30 L31 A20 A21 A22 A23 A24 A25 A26 A27 | L36 L37 L38 L39 | L40 L41 L42 L43 | L48 L49 L50 A36 A37 L51 L52 A38 A39 L53 L54 A40 L55 A41 L56 A42 A43 L57 | L58 L59 L60 L61 | L62 L63 L64 L65 makes body 2 at (25, 48.6667, 11.6667) makes body 3 at (19.4892, 29.3333, 61.1579) makes body 4 at (-30, 29.3333, -33.3333) makes body 5 at (-20, 48.6667, 8.3333) makes body 6 at (-19.4892, 29.3333, 61.1579) makes body 7 at (35, 29.3333, -21.6667) in component "Component'"
extrude "Extrude1'" add sketch "Sketch1 (2)" along normal blind 60 separate body contours L7 L17 L18 A44 L67 A46 A47 | L6 L17 L18 A44 L66 A45 A47 | L7 L15 L16 L18 L19 | L7 L10 L11 L13 A12 A13 A14 L15 L16 L19 | L6 L15 L16 L18 L19 | L6 L10 L12 L14 A9 A10 A11 L15 L16 L19 makes body 8 in component "Component'"
sketch "Sketch2" plane through (40, 0, 0) normal (1, 0, 0) x (0, 0, -1) in component "Component'"
  line L0 (-88, 10) -> (90, 10)
  line L1 (90, 10) -> (90, 70)
  line L2 (90, 70) -> (-88, 70)
  line L3 (-88, 70) -> (-88, 10)
  line L4 (-95.3524, 10) -> (104.6476, 10)
  line L5 (104.6476, 10) -> (104.6476, 65)
  line L6 (104.6476, 65) -> (-95.3524, 65)
  line L7 (-95.3524, 65) -> (-95.3524, 10)
  dimension "d40" = 200
  dimension "d41" = 55
  constraint horizontal L4
  constraint vertical L5
  constraint horizontal L6
  constraint vertical L7
  measures "d40" distance of L4.start L4.end
  measures "d41" distance of L4.start L6.end
extrude "Extrude3" cut sketch "Sketch2" against normal blind 120 contours L0 L1 L3 L4 L6 | L3 L4 L6 L7 | L1 L4 L5 L6 bodies 2 3 4 5 6 7 8 in component "Component'"
extrude "Extrude4" add sketch "Sketch1 (2)" along normal blind 60 separate body contours A8 | A15 | A16 | A17 | A18 | A19 makes body 9 at (28.0248, 50, -82.4978) makes body 10 at (36.8302, 50, 78.7861) makes body 11 at (-37.9752, 50, 17.5022) makes body 12 at (28.0248, 50, 17.5022) makes body 13 at (-29.5088, 50, 85.5793) makes body 14 at (-29.5088, 50, -78.4207) in component "Component'"
ref_plane "WorkPlane1" through (0, 67.5, 75.4003) normal (0, 0, 1) x (1, 0, 0) in component "Component'"
sketch "Sketch4" plane through (0, 67.5, 75.4003) normal (0, 0, 1) x (1, 0, 0) in component "Component'"
  line L0 (-33, 0) -> (32.8247, 0)
  line L1 (32.8247, 0) -> (32.8247, -57.541)
  line L2 (32.8247, -57.541) -> (-33, -57.541)
  line L3 (-33, -57.541) -> (-33, 0)
  circle A0 centre (0, -25) radius 20
  dimension "d47" = 40
  constraint horizontal L0
  constraint vertical L1
  constraint horizontal L2
  constraint vertical L3
  measures "d47" diameter of A0
extrude "Extrude5" add sketch "Sketch4" along normal blind 1.6 separate body makes body 15 in component "Component'"
sketch "Sketch5" plane through (0, 70, 0) normal (0, 1, 0) x (-1, 0, 0) in component "Component'"
  circle A0 centre (33, 82) radius 5
  circle A1 centre (33, 82) radius 5.5
  circle A2 centre (33, 82) radius 1
  spline S0 degree 5 poles (33.8119, 81.4162) (33.7795, 81.233) (33.7145, 80.8824) (33.6171, 80.4047) (33.4872, 79.8652) (33.3248, 79.3647) (33.1624, 79.0534) (33, 78.9469) (32.8376, 79.0534) (32.6752, 79.3647) (32.5128, 79.8652) (32.3829, 80.4047) (32.2855, 80.8824) (32.2206, 81.233) (32.1881, 81.4162) knots 0 0 0 0 0 0 0.1 0.2 0.3 0.4 0.5 0.6 0.7 0.8 0.9 1 1 1 1 1 1
  spline S1 degree 5 poles (33.5838, 82.8119) (33.767, 82.7795) (34.1176, 82.7145) (34.5953, 82.6171) (35.1348, 82.4872) (35.6353, 82.3248) (35.9466, 82.1624) (36.0531, 82) (35.9466, 81.8376) (35.6353, 81.6752) (35.1348, 81.5128) (34.5953, 81.3829) (34.1176, 81.2855) (33.767, 81.2206) (33.5838, 81.1881) knots 0 0 0 0 0 0 0.1 0.2 0.3 0.4 0.5 0.6 0.7 0.8 0.9 1 1 1 1 1 1
  spline S2 degree 5 poles (32.1881, 82.5838) (32.2206, 82.767) (32.2855, 83.1176) (32.3829, 83.5953) (32.5128, 84.1348) (32.6752, 84.6353) (32.8376, 84.9466) (33, 85.0531) (33.1624, 84.9466) (33.3248, 84.6353) (33.4872, 84.1348) (33.6171, 83.5953) (33.7145, 83.1176) (33.7795, 82.767) (33.8119, 82.5838) knots 0 0 0 0 0 0 0.1 0.2 0.3 0.4 0.5 0.6 0.7 0.8 0.9 1 1 1 1 1 1
  spline S3 degree 5 poles (32.4162, 81.1881) (32.233, 81.2206) (31.8824, 81.2855) (31.4047, 81.3829) (30.8652, 81.5128) (30.3647, 81.6752) (30.0534, 81.8376) (29.9469, 82) (30.0534, 82.1624) (30.3647, 82.3248) (30.8652, 82.4872) (31.4047, 82.6171) (31.8824, 82.7145) (32.233, 82.7795) (32.4162, 82.8119) knots 0 0 0 0 0 0 0.1 0.2 0.3 0.4 0.5 0.6 0.7 0.8 0.9 1 1 1 1 1 1
  point P0 (33, 79)
  point P1 (36, 82)
  point P2 (33, 85)
  point P3 (30, 82)
  dimension "d50" = 11
  dimension "d51" = 2
  dimension "d53" = 360
  constraint concentric A0 A1
  constraint concentric A0 A2
  constraint coincident A2 S0.start
  constraint coincident A2 S0.end
  measures "d50" diameter of A1
  measures "d51" diameter of A2
extrude "Extrude7" add sketch "Sketch5" along normal blind 2 separate body contours A0 | A1 makes body 16 in component "Component'"
extrude "Extrude6" add sketch "Sketch5" along normal blind 2 separate body contours A0 | A1 | A2 S0 S1 S2 | A2 S1 S2 S3 | A2 S0 S1 S3 | A2 S0 S2 S3 makes body 17 in component "Component'"
extrude "Extrude8" add 1 faces at (-35.0904, 72, 79.8056) along direction (0, 1, 0) blind 1 on bodies 16 bodies 16 17 in component "Component'"
extrude "Extrude9" add sketch "Sketch5" along normal blind 1 separate body contours A2 makes body 18 in component "Component'"
fillet "Fillet1" radius 1.5 1 faces at (-38.4727, 71, 81.4524) on bodies 16 in component "Component'"
mirror "Mirror1" about plane through (0, 0, 0) normal (1, 0, 0) of bodies 18 16 makes body 19 at (27.6963, 71.7841, 80.6495) makes body 20 at (32.5256, 70, 81.7774) in component "Component'"
mirror "Mirror2" about plane through (0, 0, 0) normal (0, 0, 1) of bodies 19 16 20 makes body 21 at (-27.6963, 71.7841, -80.6495) makes body 22 at (27.6963, 71.7841, -80.6495) makes body 23 at (32.5256, 70, -81.7774) in component "Component'"
copy_body "CopyPasteBodies1" bodies 18 19 16 makes body 24 makes body 25 makes body 26 in component "Component'"
move_body "Move1" bodies 24 25 26 to x (1, 0, 0) y (0, 1, 0) z (0, 0, 1) at (0, 0, -64) in component "Component'"
sketch "Sketch1 (3)" plane through (0, 10, 0) normal (0, 1, 0) x (-1, 0, 0) in component "Component''"
  arc A0 (-164.8811, -49.4467) -> (-179.5589, -130.3693) centre (-200.2067, -84.8317) ccw
  spline S0 degree 5 poles (-179.5589, -130.3693) (-178.279, -129.6405) (-176.9894, -128.9214) (-175.6902, -128.2119) (-174.3812, -127.5121) (-173.0625, -126.8221) knots 0 0 0 0 0 0 0.066925 0.066925 0.066925 0.066925 0.066925 0.066925
  spline S1 degree 5 poles (-173.0625, -126.8221) (-172.4108, -126.4811) (-169.779, -125.1187) (-165.1015, -122.8003) (-158.2442, -119.6597) (-148.9906, -115.9128) (-137.8023, -112.0905) (-126.0755, -108.8054) (-113.8059, -106.0617) (-101.0284, -103.8246) (-87.7873, -102.05) (-76.857, -100.967) (-68.4818, -100.3317) (-62.8209, -99.9855) (-59.9711, -99.8317) knots 0.066925 0.066925 0.066925 0.066925 0.066925 0.066925 0.1 0.2 0.3 0.4 0.5 0.6 0.7 0.8 0.9 1 1 1 1 1 1
  spline S2 degree 5 poles (-59.9711, -99.8317) (-57.5722, -100.2237) (-52.7745, -100.9735) (-45.578, -101.9954) (-35.9826, -103.1493) (-23.9884, -104.2199) (-11.9942, -104.8857) (0, -105.1137) (11.9942, -104.8857) (23.9884, -104.2199) (35.9826, -103.1493) (45.578, -101.9954) (52.7745, -100.9735) (57.5722, -100.2237) (59.9711, -99.8317) knots -1 -1 -1 -1 -1 -1 -0.9 -0.8 -0.7 -0.6 -0.5 -0.4 -0.3 -0.2 -0.1 0 0 0 0 0 0
  spline S3 degree 5 poles (59.9711, -99.8317) (62.8209, -99.9855) (68.4818, -100.3317) (76.857, -100.967) (87.7873, -102.05) (101.0284, -103.8246) (113.8059, -106.0617) (126.0755, -108.8054) (137.8023, -112.0905) (148.9906, -115.9128) (158.2442, -119.6597) (165.1015, -122.8003) (169.779, -125.1187) (172.4108, -126.4811) (173.0625, -126.8222) knots -1 -1 -1 -1 -1 -1 -0.9 -0.8 -0.7 -0.6 -0.5 -0.4 -0.3 -0.2 -0.1 -0.066925 -0.066925 -0.066925 -0.066925 -0.066925 -0.066925
  spline S4 degree 5 poles (173.0625, -126.8222) (174.3813, -127.5122) (175.6902, -128.2119) (176.9894, -128.9214) (178.279, -129.6405) (179.5589, -130.3693) knots -0.066925 -0.066925 -0.066925 -0.066925 -0.066925 -0.066925 0 0 0 0 0 0
  arc A1 (179.5589, -130.3693) -> (164.8811, -49.4467) centre (200.2067, -84.8317) ccw
  spline S5 degree 5 poles (164.8811, -49.4467) (163.5288, -50.018) (160.7538, -51.1452) (156.3792, -52.7897) (150.1158, -54.8884) (141.5256, -57.3456) (132.1253, -59.6259) (121.8831, -61.7224) (110.8317, -63.6422) (99.042, -65.4008) (86.5906, -67.0149) (76.1522, -68.202) (68.0735, -69.0377) (62.5785, -69.571) (59.8037, -69.8317) knots 0 0 0 0 0 0 0.1 0.2 0.3 0.4 0.5 0.6 0.7 0.8 0.9 1 1 1 1 1 1
  line L0 (59.8037, -69.8317) -> (55, -69.8317)
  arc A2 (50, -64.8317) -> (55, -69.8317) centre (55, -64.8317) ccw
  line L1 (50, -64.8317) -> (50, 64.8317)
  arc A3 (55, 69.8317) -> (50, 64.8317) centre (55, 64.8317) ccw
  line L2 (55, 69.8317) -> (59.8037, 69.8317)
  spline S6 degree 5 poles (59.8037, 69.8317) (62.5785, 69.571) (68.0735, 69.0377) (76.1522, 68.202) (86.5906, 67.0149) (99.042, 65.4008) (110.8317, 63.6422) (121.8831, 61.7224) (132.1253, 59.6259) (141.5256, 57.3456) (150.1158, 54.8884) (156.3792, 52.7897) (160.7538, 51.1452) (163.5288, 50.018) (164.8811, 49.4467) knots -1 -1 -1 -1 -1 -1 -0.9 -0.8 -0.7 -0.6 -0.5 -0.4 -0.3 -0.2 -0.1 0 0 0 0 0 0
  arc A4 (164.8811, 49.4467) -> (179.5589, 130.3693) centre (200.2067, 84.8317) ccw
  spline S7 degree 5 poles (179.5589, 130.3693) (178.279, 129.6405) (176.9894, 128.9214) (175.6902, 128.2119) (174.3813, 127.5122) (173.0625, 126.8222) knots 0 0 0 0 0 0 0.066925 0.066925 0.066925 0.066925 0.066925 0.066925
  spline S8 degree 5 poles (173.0625, 126.8222) (172.4108, 126.4811) (169.779, 125.1187) (165.1015, 122.8003) (158.2442, 119.6597) (148.9906, 115.9128) (137.8023, 112.0905) (126.0755, 108.8054) (113.8059, 106.0617) (101.0284, 103.8246) (87.7873, 102.05) (76.857, 100.967) (68.4818, 100.3317) (62.8209, 99.9855) (59.9711, 99.8317) knots 0.066925 0.066925 0.066925 0.066925 0.066925 0.066925 0.1 0.2 0.3 0.4 0.5 0.6 0.7 0.8 0.9 1 1 1 1 1 1
  spline S9 degree 5 poles (59.9711, 99.8317) (57.5722, 100.2237) (52.7745, 100.9735) (45.578, 101.9954) (35.9826, 103.1493) (23.9884, 104.2199) (11.9942, 104.8857) (0, 105.1137) (-11.9942, 104.8857) (-23.9884, 104.2199) (-35.9826, 103.1493) (-45.578, 101.9954) (-52.7745, 100.9735) (-57.5722, 100.2237) (-59.9711, 99.8317) knots 0 0 0 0 0 0 0.1 0.2 0.3 0.4 0.5 0.6 0.7 0.8 0.9 1 1 1 1 1 1
  spline S10 degree 5 poles (-59.9711, 99.8317) (-62.8209, 99.9855) (-68.4818, 100.3317) (-76.857, 100.967) (-87.7873, 102.05) (-101.0284, 103.8246) (-113.8059, 106.0617) (-126.0755, 108.8054) (-137.8023, 112.0905) (-148.9906, 115.9128) (-158.2442, 119.6597) (-165.1015, 122.8003) (-169.779, 125.1187) (-172.4108, 126.4811) (-173.0625, 126.8222) knots -1 -1 -1 -1 -1 -1 -0.9 -0.8 -0.7 -0.6 -0.5 -0.4 -0.3 -0.2 -0.1 -0.066925 -0.066925 -0.066925 -0.066925 -0.066925 -0.066925
  spline S11 degree 5 poles (-173.0625, 126.8222) (-174.3813, 127.5122) (-175.6902, 128.2119) (-176.9894, 128.9214) (-178.279, 129.6405) (-179.5589, 130.3693) knots -0.066925 -0.066925 -0.066925 -0.066925 -0.066925 -0.066925 0 0 0 0 0 0
  arc A5 (-179.5589, 130.3693) -> (-164.8811, 49.4467) centre (-200.2067, 84.8317) ccw
  spline S12 degree 5 poles (-164.8811, 49.4467) (-163.5288, 50.018) (-160.7538, 51.1452) (-156.3792, 52.7897) (-150.1158, 54.8884) (-141.5256, 57.3456) (-132.1253, 59.6259) (-121.8831, 61.7224) (-110.8317, 63.6422) (-99.042, 65.4008) (-86.5906, 67.0149) (-76.1522, 68.202) (-68.0735, 69.0377) (-62.5785, 69.571) (-59.8037, 69.8317) knots 0 0 0 0 0 0 0.1 0.2 0.3 0.4 0.5 0.6 0.7 0.8 0.9 1 1 1 1 1 1
  line L3 (-59.8037, 69.8317) -> (-55, 69.8317)
  arc A6 (-50, 64.8317) -> (-55, 69.8317) centre (-55, 64.8317) ccw
  line L4 (-50, 64.8317) -> (-50, -64.8317)
  arc A7 (-55, -69.8317) -> (-50, -64.8317) centre (-55, -64.8317) ccw
  line L5 (-55, -69.8317) -> (-59.8037, -69.8317)
  spline S13 degree 5 poles (-59.8037, -69.8317) (-62.5785, -69.571) (-68.0735, -69.0377) (-76.1522, -68.202) (-86.5906, -67.0149) (-99.042, -65.4008) (-110.8317, -63.6422) (-121.8831, -61.7224) (-132.1253, -59.6259) (-141.5256, -57.3456) (-150.1158, -54.8884) (-156.3792, -52.7897) (-160.7538, -51.1452) (-163.5288, -50.018) (-164.8811, -49.4467) knots -1 -1 -1 -1 -1 -1 -0.9 -0.8 -0.7 -0.6 -0.5 -0.4 -0.3 -0.2 -0.1 0 0 0 0 0 0
  circle A8 centre (200.2067, -84.8317) radius 40
  circle A9 centre (200.2067, -84.8317) radius 10
  circle A10 centre (200.2067, -84.8317) radius 25
  line L6 (204.9024, -45.1083) -> (204.9024, -60.2767)
  line L7 (194.9698, -60.3864) -> (194.9698, -45.176)
  line L8 (168.1531, -60.9033) -> (181.2893, -68.4875)
  line L9 (176.4179, -77.1442) -> (163.2454, -69.5391)
  line L10 (163.4573, -100.6268) -> (176.5935, -93.0426)
  line L11 (181.6547, -101.5896) -> (168.4822, -109.1948)
  line L12 (195.5109, -124.5551) -> (195.5109, -109.3868)
  line L13 (205.4435, -109.2771) -> (205.4435, -124.4874)
  line L14 (232.2602, -108.7601) -> (219.124, -101.1759)
  line L15 (223.9954, -92.5192) -> (237.1679, -100.1244)
  line L16 (236.956, -69.0367) -> (223.8198, -76.6209)
  line L17 (218.7586, -68.0738) -> (231.9311, -60.4687)
  circle A11 centre (200.2067, -84.8317) radius 2.5
  circle A12 centre (200.2067, -84.8317) radius 35
  circle A13 centre (200.2067, -84.8317) radius 40.5
  dimension "d68" = 80
  dimension "d71" = 20
  dimension "d72" = 50
  dimension "d76" = 360
  dimension "d77" = 5
  dimension "d91" = 70
  dimension "d121" = 81
  constraint concentric A1 A8
  constraint concentric A1 A9
  constraint concentric A8 A10
  constraint vertical L6
  constraint vertical L7
  constraint coincident A8 L7.end
  constraint coincident A10 L6.end
  constraint coincident A10 L7.start
  constraint coincident A8 L6.start
  constraint concentric A8 A11
  constraint concentric A11 A12
  constraint concentric A8 A13
  measures "d68" diameter of A8
  measures "d71" diameter of A9
  measures "d72" diameter of A10
  measures "d77" diameter of A11
  measures "d91" diameter of A12
  measures "d121" diameter of A13
extrude "Extrude15" add sketch "Sketch1 (3)" along normal blind 20 separate body contours A13 makes body 27 in component "Component''"
extrude "Extrude8'" add sketch "Sketch1 (3)" along normal blind 70 separate body contours A11 makes body 28 in component "Component''"
extrude "Extrude5'" add sketch "Sketch1 (3)" along normal blind 70 separate body contours A9 makes body 29 in component "Component''"
extrude "Extrude4'" add sketch "Sketch1 (3)" along normal blind 30 separate body contours A8 L16 L17 A12 | A8 L14 L15 A12 | A10 L16 L17 A12 | A10 L14 L15 A12 | A8 L6 L7 A12 | A8 L12 L13 A12 | A10 L6 L7 A12 | A10 L12 L13 A12 | A8 L8 L9 A12 | A8 L10 L11 A12 | A10 L8 L9 A12 | A10 L10 L11 A12 makes body 30 at (-228.3862, 20, -95.0543) makes body 31 at (-172.0271, 30, -74.6092) makes body 32 at (-205.4435, 20, -114.3472) makes body 33 at (-223.1494, 20, -65.5388) makes body 34 at (-194.9698, 20, -55.3162) makes body 35 at (-177.2639, 30, -104.1247) in component "Component''"
extrude "Extrude2'" add sketch "Sketch1 (3)" along normal blind 40 separate body contours A10 makes body 36 in component "Component''"
extrude "Extrude1''" add sketch "Sketch1 (3)" along normal blind 20 separate body contours A8 L15 L16 A12 | A8 L16 L17 A12 | A8 L14 L15 A12 | A8 L6 L17 A12 | A10 L16 L17 A12 | A8 L13 L14 A12 | A10 L14 L15 A12 | A8 L6 L7 A12 | A10 | A8 L12 L13 A12 | A8 L7 L8 A12 | A10 L6 L7 A12 | A8 L11 L12 A12 | A10 L12 L13 A12 | A8 L8 L9 A12 | A8 L10 L11 A12 | A8 L9 L10 A12 | A10 L8 L9 A12 | A10 L10 L11 A12 makes body 37 in component "Component''"
sketch "Sketch2 (2)" plane through (0, 0, 0) normal (0, 0, 1) x (1, 0, 0) in component "Component''"
  line L0 (-240, 10) -> (-160, 10)
  line L1 (-200, 10) -> (-200, 62.3515)
  line L2 (-240, 30) -> (-160, 30)
  constraint horizontal L0
  constraint midpoint L0 L1.start
  constraint perpendicular L0 L1
  constraint perpendicular L1 L2
sketch "Sketch3" plane through (0, 0, 0) normal (0, 0, 1) x (1, 0, 0) in component "Component''"
  line L0 (-226.0577, 40.2115) -> (-175, 40.2115)
  line L1 (-175, 40.2115) -> (-175, 30.2115)
  line L2 (-175, 30.2115) -> (-226.0577, 30.2115)
  line L3 (-226.0577, 30.2115) -> (-226.0577, 40.2115)
  dimension "d80" = 10
  constraint horizontal L0
  constraint vertical L1
  constraint horizontal L2
  constraint vertical L3
  measures "d80" distance of L0.start L2.end
extrude "Extrude3'" cut sketch "Sketch3" against normal blind 205 bodies 36 makes body 38 at (-225.0824, 23.4744, -82.3425) in component "Component''"
chamfer "Chamfer1" distance 15 angle 45 1 edges at (-234.7106, 40, -64.5961) on bodies 33 in component "Component''"
chamfer "Chamfer2" distance 15 angle 45 1 edges at (-199.934, 40, -44.8326) on bodies 34 in component "Component''"
chamfer "Chamfer3" distance 15 angle 45 1 edges at (-165.4301, 40, -65.0683) on bodies 31 in component "Component''"
chamfer "Chamfer4" distance 15 angle 45 1 edges at (-165.7027, 40, -105.0674) on bodies 35 in component "Component''"
chamfer "Chamfer5" distance 15 angle 45 1 edges at (-200.4793, 40, -124.8308) on bodies 32 in component "Component''"
chamfer "Chamfer6" distance 15 angle 45 1 edges at (-234.9832, 40, -104.5952) on bodies 30 in component "Component''"
sketch "Sketch4 (2)" plane through (0, 50, 0) normal (0, 1, 0) x (-1, 0, 0) in component "Component''"
  circle A0 centre (200.2067, -84.8317) radius 10
  circle A1 centre (200.2067, -84.8317) radius 25
  circle A2 centre (200.0841, -102.1381) radius 5
  circle A3 centre (217.513, -84.9543) radius 5
  circle A4 centre (200.3292, -67.5254) radius 5
  circle A5 centre (182.9003, -84.7091) radius 5
  dimension "d92" = 10
  dimension "d94" = 360
  measures "d92" diameter of A2
sketch "Sketch5 (2)" plane through (0, 0, 0) normal (0, 0, 1) x (1, 0, 0) in component "Component''"
  line L0 (-211.0791, 60) -> (-190, 60)
  line L1 (-190, 60) -> (-190, 50)
  line L2 (-190, 50) -> (-211.0791, 50)
  line L3 (-211.0791, 50) -> (-211.0791, 60)
  constraint horizontal L0
  constraint vertical L1
  constraint horizontal L2
  constraint vertical L3
extrude "Extrude6'" cut sketch "Sketch5 (2)" against normal blind 205 bodies 29 makes body 39 at (-210.157, 36.6667, -83.836) in component "Component''"
extrude "Extrude7'" cut sketch "Sketch4 (2)" against normal blind 5 contours A2 | A3 | A4 | A5 bodies 36 in component "Component''"
pipe "Pipe1" add diameter 2 along 1 edges at (-190.2067, 60, -84.8317) on bodies 29 bodies 29 in component "Component''"
ref_plane "WorkPlane1" through (-200.2067, 80.9105, -74.8317) normal (0, 0, 1) x (-1, 0, 0) in component "Component''"